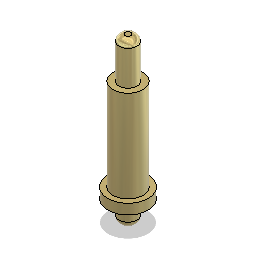
Anschluss-Element v11 (Autodesk Fusion 360 archive; units mm, degrees)
design "Pogo-Pin"
Autodesk Fusion 360 part; units mm, degrees
sketch "Skizze1" plane through (0, 0, 0) normal (0, 1, 0) x (1, 0, 0)
  circle A0 centre (0, 0) radius 0.99
  circle A1 centre (0, 0) radius 0.44
  circle A2 centre (0, 0) radius 0.735
  dimension "d1" = 1.98
  dimension "d2" = 0.88
  dimension "d3" = 1.47
  constraint coincident A0.centre A1.centre
  constraint concentric A0 A2
  measures "d1" diameter of A0
  measures "d2" diameter of A1
  measures "d3" diameter of A2
extrude "Extrusion1" add sketch "Skizze1" against normal blind 0.5 contours A0 | A1 | A2 makes body 1
extrude "Extrusion2" add sketch "Skizze1" along normal blind 4.5 contours A2 bodies 1
extrude "Extrusion3" add sketch "Skizze1" against normal blind 1.5 separate body contours A1 makes body 2
extrude "Extrusion4" add sketch "Skizze1" along normal blind 6.5 and the other way blind -2.3 separate body contours A1 makes body 3
fillet "Abrundung1" radius 0.3 1 edges at (-0.4102, 6.5, 0.1591) on bodies 3
fillet "Abrundung2" radius 0.3 1 edges at (-0.4102, -1.5, -0.1591) on bodies 2
equation "d6 = 5 mm - 0.5 mm"
named bodies: "Hülse (1)", "Anschluss", "Pin"
